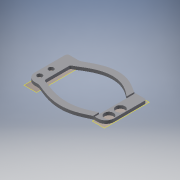
# Autodesk Inventor part: 28_Objectholder
Saved by Autodesk Inventor 2016 (Build 200138000, 138)
## iProperties
Created: 2016-12-20
Part Number: 28_Objectholder
Material: Generisch
Document SubType Name: Modeling
Designer: diederichbenedict
Density: 1 g/cm^3
Appearance: Vorgabe
Author: diederichbenedict
Autodesk Inventor part; units mm, degrees
ref_plane "YZ Plane" through (0, 0, 0) normal (1, 0, 0) x (0, 1, 0)
ref_plane "XZ Plane" through (0, 0, 0) normal (0, 1, 0) x (-1, 0, 0)
ref_plane "XY Plane" through (0, 0, 0) normal (0, 0, 1) x (1, 0, 0)
ref_plane "Arbeitsebene1" through (0, 0, 0) normal (0, 0, 1) x (1, 0, 0)
sketch "Skizze1" plane through (0, 0, 0) normal (0, 0, 1) x (1, 0, 0)
  circle A0 centre (0.5, -12) radius 2.5 construction
  circle A1 centre (0.5, -0.7611) radius 2.5 construction
  arc A2 (-2.5, -20) -> (5.5, -12) centre (-2.5, -12) ccw construction
  line L0 (5.5, -12) -> (5.5, 20) construction
  line L1 (5.5, 20) -> (-5.5, 20) construction
  line L2 (-5.5, 20) -> (-5.5, -20) construction
  line L3 (-5.5, -20) -> (-2.5, -20) construction
  circle A3 centre (0.5, -12) radius 2.5 projected
  circle A4 centre (0.5, -0.7611) radius 2.5 projected
  arc A5 (-2.5, -20) -> (5.5, -12) centre (-2.5, -12) ccw projected
  line L4 (5.5, -12) -> (5.5, 20) projected
  line L5 (5.5, 20) -> (-5.5, 20) projected
  line L6 (-5.5, 20) -> (-5.5, -20) projected
  line L7 (-5.5, -20) -> (-2.5, -20) projected
  circle A6 centre (-67.5023, -0.7611) radius 2.5 projected
  circle A7 centre (-67.5, -12) radius 2.5 projected
  arc A8 (-72.5, -12) -> (-64.5, -20) centre (-64.5, -12) ccw projected
  line L8 (-61.25, -20) -> (-64.5, -20) projected
  line L9 (-61.25, 20) -> (-61.25, -20) projected
  line L10 (-72.5, 20) -> (-61.25, 20) projected
  line L11 (-72.5, -12) -> (-72.5, 20) projected
  line L12 (-61.25, -20) -> (-5.5, -20) construction
  line L13 (-5.5, -20) -> (-5.5, -14)
  line L14 (-5.5, -14) -> (-61.25, -14) construction
  line L15 (-61.25, -14) -> (-61.25, -20)
  line L16 (-61.25, 20) -> (-5.5, 20) construction
  line L17 (-5.5, 20) -> (-5.5, 12)
  line L18 (-5.5, 12) -> (-61.25, 12) construction
  line L19 (-61.25, 12) -> (-61.25, 20)
  circle A9 centre (-29.6976, 1.3899) radius 18 construction
  line L20 (-17.862, 21.8899) -> (-41.5333, 21.8899) construction
  line L21 (-41.5333, 21.8899) -> (-53.369, 1.3899) construction
  line L22 (-53.369, 1.3899) -> (-41.5333, -19.1101) construction
  line L23 (-41.5333, -19.1101) -> (-17.862, -19.1101) construction
  line L24 (-17.862, -19.1101) -> (-6.0263, 1.3899) construction
  line L25 (-6.0263, 1.3899) -> (-17.862, 21.8899) construction
  line L26 (-29.6976, 1.3899) -> (-29.6976, 61.6034) construction
  line L27 (-29.6976, 61.6034) -> (-29.6976, -53.0007) construction
  line L28 (-61.25, -20) -> (-55.25, -20) construction
  line L29 (-55.25, -20) -> (-29.6976, -39.6101) construction
  line L30 (-29.6976, -39.6101) -> (-11.5, -20) construction
  line L31 (-11.5, -20) -> (-5.5, -20) construction
  spline S0 degree 4 poles (-61.25, -20) (-55.25, -20) (-29.6976, -39.6101) (-11.5, -20) (-5.5, -20) knots 1 1 1 1 1 2 2 2 2 2
  line L32 (-61.25, -14) -> (-55.25, -14) construction
  line L33 (-55.25, -14) -> (-29.6976, -32.7963) construction
  line L34 (-29.6976, -32.7963) -> (-11.5, -14) construction
  line L35 (-11.5, -14) -> (-5.5, -14) construction
  spline S1 degree 4 poles (-61.25, -14) (-55.25, -14) (-29.6976, -32.7963) (-11.5, -14) (-5.5, -14) knots 1 1 1 1 1 2 2 2 2 2
  line L36 (-61.25, 12) -> (-55.25, 12) construction
  line L37 (-55.25, 12) -> (-29.6976, 42.3899) construction
  line L38 (-29.6976, 42.3899) -> (-8.7442, 12) construction
  line L39 (-8.7442, 12) -> (-5.5, 12) construction
  spline S2 degree 4 poles (-61.25, 12) (-55.25, 12) (-29.6976, 42.3899) (-8.7442, 12) (-5.5, 12) knots 1 1 1 1 1 2 2 2 2 2
  line L40 (-5.5, 20) -> (-11.5, 20) construction
  line L41 (-11.5, 20) -> (-29.6976, 46.393) construction
  line L42 (-29.6976, 46.393) -> (-55.25, 20) construction
  line L43 (-55.25, 20) -> (-61.25, 20) construction
  spline S3 degree 4 poles (-5.5, 20) (-11.5, 20) (-29.6976, 46.393) (-55.25, 20) (-61.25, 20) knots 1 1 1 1 1 2 2 2 2 2
  point P0 (0, 0)
  point P1 (-5.5, 16)
  dimension "d7" = 6
  dimension "d8" = 8
  dimension "d15" = 6
  dimension "d16" = 6
  constraints: 20 end point, 15 point on line, 5 parallel, 3 collinear, 3 perpendicular, 2 horizontal, 1 midpoint, 1 vertical, 12 other
  measures "d7" distance of L13.end L12.end
  measures "d8" distance of L16.end L17.end
  measures "d15" distance of L30.end L2.end
  measures "d16" distance of L8.start L28.end
extrude "Extrusion1" add sketch "Skizze1" along normal blind 3 contours L7 L6 L5 L4 A5 | S0 L9 S1 L6 | L8 A8 L11 L10 L9 | L6 S2 L9 S3
sketch "Skizze2" plane through (0, 0, 3) normal (0, 0, 1) x (1, 0, 0)
  circle A0 centre (0.5, -0.7611) radius 2.5 projected
  circle A1 centre (0.5, -12) radius 2.5 projected
  circle A2 centre (0.5, -0.7611) radius 4.5
  circle A3 centre (0.5, -12) radius 4.5
  point P0 (0, 0)
  dimension "d2" = 2
  dimension "d3" = 2
  constraints: 2 centre point
  measures "d2" radial gap between concentric circles of A0 A2
  measures "d3" radial gap between concentric circles of A1 A3
extrude "Extrusion2" cut sketch "Skizze2" against normal blind 3
ref_plane "Arbeitsebene2" through (-66.5374, 1.3229, -3) normal (0, 0, 1) x (1, 0, 0)
sketch "Skizze3" plane through (-64.5, -20, 0) normal (0, -1, 0) x (1, 0, 0)
  line L0 (59, 0) -> (62, 0) projected
  line L1 (62, 0) -> (62, 3) projected
  line L2 (59, 3) -> (62, 3) projected
  line L3 (60.5, 1) -> (69.5, 1) projected
  line L4 (62, 3) -> (60.5, 3)
  line L5 (60.5, 3) -> (60.5, 1)
  line L6 (60.5, 1) -> (62, 1)
  line L7 (62, 1) -> (62, 3)
  line L8 (59, 3) -> (57.5, 3)
  line L9 (57.5, 3) -> (57.5, 1)
  line L10 (57.5, 1) -> (59, 1)
  line L11 (59, 1) -> (59, 3)
  line L12 (59, 0) -> (59, 3) projected
  point P0 (64.5, 0)
  dimension "d13" = 1.5
  dimension "d14" = 1
  constraints: 16 end point, 4 parallel, 2 horizontal, 2 perpendicular
  measures "d13" distance of L10.end L9.end
  measures "d14" distance between parallel lines of L10 L0
extrude "Extrusion3" cut sketch "Skizze3" against normal through all contours L10 L9 L8 L11
fillet "Rundung1" [suppressed]
fillet "Rundung2" radius 2 4 edges at (-61.25, 12, 1.5) (-61.25, -14, 1.5) (5.5, 20, 1.5) (-72.5, 20, 1.5)
